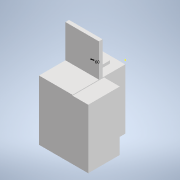
# Autodesk Inventor part: CMM
Saved by Autodesk Inventor 2020 (Build 240168000, 168)
## iProperties
Created: 2019-10-05
Part Number: CMM
Material: Genérico
Document SubType Name: Modeling
Designer: dasa1
Density: 1 g/cm^3
Appearance: Valor por defecto
Author: dasa1
Autodesk Inventor part; units mm, degrees
ref_plane "YZ Plane" through (0, 0, 0) normal (1, 0, 0) x (0, 1, 0)
ref_plane "XZ Plane" through (0, 0, 0) normal (0, 1, 0) x (-1, 0, 0)
ref_plane "XY Plane" through (0, 0, 0) normal (0, 0, 1) x (1, 0, 0)
sketch "Boceto1" plane through (0, 0, 0) normal (0, 1, 0) x (-1, 0, 0)
  line L0 (0, 0) -> (640, 0)
  line L1 (640, 0) -> (640, 1009)
  line L2 (640, 1009) -> (0, 1009)
  line L3 (0, 1009) -> (0, 0)
  dimension "d0" = 640
  dimension "d1" = 1009
  constraints: 8 end point, 2 parallel, 1 horizontal, 1 perpendicular
  measures "d0" distance of L2.end L1.end
  measures "d1" distance of L1.end L0.end
extrude "Extrusión1" add sketch "Boceto1" along normal blind 1147
sketch "Boceto2" plane through (0, 1147, 0) normal (0, 1, 0) x (1, 0, 0)
  line L0 (-640, 0) -> (-640, -1009) construction
  line L1 (-640, -1009) -> (0, -1009) construction
  line L2 (0, -1009) -> (0, 0) construction
  line L3 (0, 0) -> (-640, 0) construction
  line L4 (-640, 0) -> (-640, -1009) construction
  line L5 (-640, -1009) -> (-640, -504.5) construction
  line L6 (0, -1009) -> (0, 0) construction
  line L7 (-640, -504.5) -> (0, -504.5) construction
  line L8 (0, -504.5) -> (0, -434.5) construction
  line L9 (0, -434.5) -> (-640, -434.5) construction
  line L10 (-640, -434.5) -> (-640, -504.5) construction
  line L11 (0, -434.5) -> (-640, -434.5)
  line L12 (-640, -434.5) -> (-640, -504.5)
  line L13 (-640, -504.5) -> (0, -504.5)
  line L14 (0, -504.5) -> (0, -434.5)
  dimension "d4" = 504.5
  dimension "d5" = 70
  dimension "d6" = 70
  constraints: 18 end point, 4 parallel, 2 horizontal, 2 perpendicular, 2 point on line, 1 midpoint
  measures "d4" distance of L0.end L5.end
  measures "d5" distance of L8.end L7.end
  measures "d6" distance of L12.end L11.end
extrude "Extrusión2" add sketch "Boceto2" along normal blind 633
sketch "Boceto3" plane through (0, 1147, 0) normal (0, 1, 0) x (1, 0, 0)
  line L0 (-640, -434.5) -> (0, -434.5) construction
  line L1 (0, -434.5) -> (0, 0) construction
  line L2 (0, 0) -> (-640, 0) construction
  line L3 (-640, 0) -> (-640, -434.5) construction
  line L4 (0, -434.5) -> (0, 0) construction
  line L5 (0, -434.5) -> (-160, -434.5) construction
  line L6 (0, -434.5) -> (-640, -434.5) construction
  line L7 (-640, -434.5) -> (-640, -504.5) construction
  line L8 (-640, -434.5) -> (-480, -434.5) construction
  line L9 (-480, -434.5) -> (-160, -434.5)
  line L10 (-160, -434.5) -> (-160, -134.5)
  line L11 (-160, -134.5) -> (-480, -134.5)
  line L12 (-480, -134.5) -> (-480, -434.5)
  dimension "d9" = 160
  dimension "d10" = 160
  dimension "d11" = 300
  constraints: 12 end point, 2 parallel, 2 point on line, 1 horizontal, 1 perpendicular
  measures "d9" distance of L0.end L5.end
  measures "d10" distance of L0.start L8.end
  measures "d11" distance of L10.end L9.end
extrude "Extrusión3" add sketch "Boceto3" along normal blind 53
sketch "Boceto4" plane through (0, 1200, 0) normal (0, 1, 0) x (1, 0, 0)
  line L0 (-160, -434.5) -> (-480, -434.5) construction
  line L1 (-160, -434.5) -> (-160, -134.5) construction
  line L2 (-160, -134.5) -> (-480, -134.5) construction
  line L3 (-480, -134.5) -> (-480, -434.5) construction
  line L4 (0, -434.5) -> (-640, -434.5) construction
  line L5 (-320, -434.5) -> (-320, -309.5) construction
  circle A0 centre (-320, -309.5) radius 30 construction
  line L6 (-320, -309.5) -> (-395, -309.5) construction
  line L7 (-395, -309.5) -> (-395, -339.5) construction
  line L8 (-395, -339.5) -> (-320, -339.5) construction
  line L9 (-320, -339.5) -> (-320, -309.5) construction
  line L10 (-395, -339.5) -> (-245, -339.5)
  line L11 (-245, -339.5) -> (-245, -279.5)
  line L12 (-245, -279.5) -> (-395, -279.5)
  line L13 (-395, -279.5) -> (-395, -339.5)
  point P0 (0, 0)
  dimension "d14" = 125
  dimension "d15" = 60
  dimension "d16" = 75
  dimension "d17" = 30
  dimension "d18" = 150
  dimension "d19" = 60
  constraints: 18 end point, 4 parallel, 2 horizontal, 2 perpendicular, 1 centre point, 1 coincident, 1 midpoint, 1 vertical
  measures "d14" distance of L5.start L5.end
  measures "d15" diameter of A0
  measures "d16" distance of L8.end L7.end
  measures "d17" distance of L7.end L6.end
  measures "d18" distance of L12.end L11.end
  measures "d19" distance of L11.end L10.end
extrude "Extrusión4" add sketch "Boceto4" along normal blind 20
sketch "Boceto5" plane through (0, 1220, 0) normal (0, 1, 0) x (1, 0, 0)
  line L0 (-245, -279.5) -> (-395, -279.5) construction
  line L1 (-395, -279.5) -> (-395, -339.5) construction
  line L2 (-395, -339.5) -> (-245, -339.5) construction
  line L3 (-245, -339.5) -> (-245, -279.5) construction
  circle A0 centre (-320, -309.5) radius 30 construction
  line L4 (-320, -309.5) -> (-352, -309.5) construction
  line L5 (-352, -309.5) -> (-288, -309.5) construction
  line L6 (-395, -339.5) -> (-245, -339.5) projected
  line L7 (-352, -339.5) -> (-395, -339.5)
  line L8 (-395, -339.5) -> (-395, -279.5)
  line L9 (-395, -279.5) -> (-352, -279.5)
  line L10 (-352, -279.5) -> (-352, -339.5)
  line L11 (-245, -279.5) -> (-245, -339.5) projected
  line L12 (-395, -279.5) -> (-245, -279.5) projected
  line L13 (-245, -339.5) -> (-288, -339.5)
  line L14 (-288, -339.5) -> (-288, -279.5)
  line L15 (-288, -279.5) -> (-245, -279.5)
  line L16 (-245, -279.5) -> (-245, -339.5)
  point P0 (0, 0)
  dimension "d22" = 60
  dimension "d23" = 32
  dimension "d24" = 64
  constraints: 20 end point, 4 parallel, 3 horizontal, 3 point on line, 2 perpendicular, 1 centre point
  measures "d22" diameter of A0
  measures "d23" distance of L4.start L4.end
  measures "d24" distance of L4.end L5.end
extrude "Extrusión5" add sketch "Boceto5" along normal blind 35 contours L8 L9 L10 L6 | L14 L12 L11 L6
chamfer "Chaflán1" distance 20 angle 45 1 edges at (-395, 1255, 309.5)
sketch "Boceto6" plane through (0, 0, 0) normal (0, -1, 0) x (1, 0, 0)
  line L0 (-640, 0) -> (-640, 1009) construction
  line L1 (0, 0) -> (-640, 0) construction
  line L2 (0, 1009) -> (0, 0) construction
  line L3 (-640, 1009) -> (0, 1009) construction
  line L4 (-640, 1009) -> (0, 1009) projected
  line L5 (0, 1009) -> (300, 1009)
  line L6 (300, 1009) -> (300, 405)
  line L7 (300, 405) -> (0, 405)
  line L8 (0, 405) -> (0, 1009)
  dimension "d30" = 300
  dimension "d31" = 604
  constraints: 8 end point, 2 parallel, 1 horizontal, 1 perpendicular
  measures "d30" distance of L6.end L7.end
  measures "d31" distance of L5.end L6.end
extrude "Extrusión6" add sketch "Boceto6" against normal blind 1133
sketch "Boceto7" plane through (0, 1220, 0) normal (0, 1, 0) x (1, 0, 0)
  line L0 (-352, -279.5) -> (-352, -339.5) projected
  line L1 (-352, -339.5) -> (-288, -339.5) projected
  line L2 (-288, -339.5) -> (-288, -279.5) projected
  line L3 (-288, -279.5) -> (-352, -279.5) projected
  circle A0 centre (-320, -309.5) radius 30
  point P0 (0, 0)
  dimension "d34" = 60
  dimension "d35" = 32
  constraints: 1 centre point, 1 coincident, 1 tangent
  measures "d34" diameter of A0
  measures "d35" distance from line of A0.centre L2
